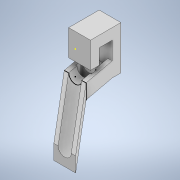
# Autodesk Inventor part: top_part
Saved by Autodesk Inventor 2021 (Build 250183000, 183)
## iProperties
Created: 2021-04-02
Part Number: top_part
Material: Generic
Document SubType Name: Modeling
Designer: Jawal
Density: 1 g/cm^3
Appearance: Default
Author: Jawal
Autodesk Inventor part; units mm, degrees
ref_plane "YZ Plane" through (0, 0, 0) normal (1, 0, 0) x (0, 1, 0)
ref_plane "XZ Plane" through (0, 0, 0) normal (0, 1, 0) x (-1, 0, 0)
ref_plane "XY Plane" through (0, 0, 0) normal (0, 0, 1) x (1, 0, 0)
sketch "Sketch1" plane through (0, 0, 0) normal (0, 0, 1) x (1, 0, 0)
  line L0 (-12.5, 12.5) -> (12.5, 12.5)
  line L1 (12.5, 12.5) -> (12.5, -37.5)
  line L2 (12.5, -37.5) -> (-12.5, -37.5)
  line L3 (-12.5, -37.5) -> (-12.5, 12.5)
  point P0 (0, 0)
  dimension "d0" = 25
  dimension "d1" = 50
  dimension "d2" = 12.5
  dimension "d3" = 12.5
  constraints: 8 end point, 2 parallel, 1 horizontal, 1 perpendicular
  measures "d0" distance of L0.start L0.end
  measures "d1" distance of L0.end L1.end
  measures "d2" distance from line of L1 point (0, 0)
  measures "d3" distance from line of point (0, 0) L0
extrude "Extrusion1" add sketch "Sketch1" along normal blind 10
sketch "Sketch2" plane through (0, 0, 0) normal (0, 0, -1) x (-1, 0, 0)
  circle A0 centre (0, -33) radius 1.5
  circle A1 centre (0, 0) radius 7.5
  dimension "d7" = 3
  dimension "d8" = 33
  dimension "d17" = 15
  constraints: 2 centre point, 1 coincident
  measures "d7" diameter of A0
  measures "d8" distance of A0.centre point (0, 0)
  measures "d17" diameter of A1
extrude "Extrusion2" add sketch "Sketch2" along normal blind 6 contours A0
sketch "Sketch3" plane through (0, 0, 10) normal (0, 0, 1) x (1, 0, 0)
  arc A0 (7.5, 0) -> (-7.5, 0) centre (0, 0) ccw
  line L0 (-7.5, 0) -> (-12.5, 0)
  line L1 (-12.5, 12.5) -> (-12.5, -37.5) projected
  line L2 (-12.5, 0) -> (-12.5, 12.5)
  line L3 (12.5, 12.5) -> (-12.5, 12.5) projected
  line L4 (12.5, 12.5) -> (12.5, 0)
  line L5 (12.5, -37.5) -> (12.5, 12.5) projected
  line L6 (7.5, 0) -> (12.5, 0)
  dimension "d11" = 15
  constraints: 8 end point, 2 point on circle, 2 point on line, 1 centre point, 1 coincident, 1 collinear, 1 horizontal, 1 perpendicular
  measures "d11" diameter of A0
extrude "Extrusion3" add sketch "Sketch3" along normal blind 15
sketch "Sketch4" plane through (0, 0, 25) normal (0, 0, 1) x (1, 0, 0)
  line L0 (-12.5, 12.5) -> (-12.5, 0) projected
  line L1 (-12.5, 12.5) -> (12.5, 12.5)
  line L2 (12.5, 12.5) -> (12.5, -17.5)
  line L3 (12.5, -17.5) -> (-12.5, -17.5)
  line L4 (-12.5, -17.5) -> (-12.5, 12.5)
  point P0 (0, 0)
  dimension "d14" = 25
  dimension "d21" = 30
  constraints: 8 end point, 2 parallel, 1 horizontal, 1 perpendicular
  measures "d14" distance of L2.end L3.end
  measures "d21" distance of L1.end L2.end
extrude "Extrusion4" add sketch "Sketch4" along normal blind 10
sketch "Sketch5" plane through (0, 0, 0) normal (0, 0, -1) x (-1, 0, 0)
  circle A0 centre (0, 0) radius 7.5
  dimension "d18" = 15
  constraints: 1 centre point, 1 coincident
  measures "d18" diameter of A0
extrude "Extrusion5" cut sketch "Sketch5" against normal blind 10
sketch "Sketch6" plane through (0, 0, 10) normal (0, 0, 1) x (1, 0, 0)
  line L0 (-12.5, -20.5) -> (-12.5, -37.5)
  line L1 (-12.5, -37.5) -> (12.5, -37.5) projected
  line L2 (-12.5, -37.5) -> (12.5, -37.5)
  line L3 (12.5, -37.5) -> (12.5, -20.5)
  line L4 (12.5, -37.5) -> (12.5, 0) projected
  arc A0 (-7.5, -20.5) -> (7.5, -20.5) centre (0, -20.5) ccw
  line L5 (-12.5, -20.5) -> (-7.5, -20.5)
  line L6 (7.5, -20.5) -> (12.5, -20.5)
  line L7 (-12.5, 0) -> (-12.5, -37.5) projected
  line L8 (-12.5, -29) -> (12.5, -29)
  point P0 (0, 0)
  dimension "d22" = 15
  dimension "d23" = 17
  dimension "d24" = 17
  constraints: 12 end point, 3 point on line, 2 horizontal, 2 point on circle, 1 centre point, 1 collinear, 1 perpendicular
  measures "d22" diameter of A0
  measures "d23" distance of L1.end L3.end
  measures "d24" distance of L0.start L0.end
ref_plane "Work Plane1" through (0, -37.5, 0) normal (-1, 0, 0) x (0, 0, 1)
sketch "Sketch8" plane through (0, -37.5, 0) normal (-1, 0, 0) x (0, 0, 1)
  line L0 (10, 0) -> (10, 37.5) projected
  line L1 (10, 8.5) -> (40, 1.574)
  line L2 (10, 8.5) -> (40.7891, 8.5) construction
  line L3 (0, 0) -> (10, 0) projected
  point P0 (0, 37.5)
  dimension "d26" = 13
  dimension "d27" = 8.5
  dimension "d32" = 30
  constraints: 4 end point, 1 equal length, 1 horizontal, 1 point on line
  measures "d26" angle of L1 L2
  measures "d27" distance between parallel lines of L3 L2
  measures "d32" distance from line of L1.end L0
sweep "Sweep1" add profiles "Sketch6" path "Sketch8" path curves L1
thread "Thread1"
sketch "Sketch9" plane through (-12.5, -44.426, 40) normal (0, 0, 1) x (1, 0, 0)
  point P0 (12.5, 44.426)
sketch "Sketch10" plane through (-12.5, -44.426, 40) normal (0, 0, 1) x (1, 0, 0)
  point P0 (12.5, 44.426)
ref_plane "Work Plane2" through (12.5, -44.426, 40) normal (0, -1, 0) x (1, 0, 0)
sketch "Sketch12" plane through (12.5, -44.426, 40) normal (0, -1, 0) x (1, 0, 0)
  line L0 (-3.5, -15.5) -> (-21.5, -15.5)
  line L1 (-21.5, -15.5) -> (-21.5, -9.5)
  line L2 (-21.5, -9.5) -> (-3.5, -9.5)
  line L3 (-3.5, -9.5) -> (-3.5, -15.5)
  line L4 (0, -30) -> (0, 0) projected
  point P0 (-12.5, -40)
  dimension "d33" = 18
  dimension "d34" = 6
  dimension "d35" = 3.5
  dimension "d36" = 14.5
  constraints: 8 end point, 1 horizontal, 1 parallel, 1 perpendicular
  measures "d33" distance of L1.end L2.end
  measures "d34" distance of L0.end L1.end
  measures "d35" distance between parallel lines of L4 L3
  measures "d36" distance from line of L4.start L0
extrude "Extrusion6" cut sketch "Sketch12" against normal blind 25
sketch "Sketch13" plane through (-12.5, -44.426, 40) normal (0, 0, 1) x (1, 0, 0)
  line L0 (5, 17) -> (0, 17) projected
  line L1 (5, 17) -> (0, 17)
  line L2 (0, 17) -> (0, 0) projected
  line L3 (0, 17) -> (0, 0)
  line L4 (0, 0) -> (25, 0) projected
  line L5 (0, 0) -> (25, 0)
  line L6 (25, 0) -> (25, 17) projected
  line L7 (25, 0) -> (25, 17)
  arc A0 (5, 17) -> (20, 17) centre (12.5, 17) ccw projected
  line L8 (25, 17) -> (20, 17)
  arc A1 (5, 17) -> (20, 17) centre (12.5, 17) ccw
  point P0 (12.5, 44.426)
  constraints: 10 end point, 2 collinear, 2 perpendicular, 2 point on circle, 1 centre point, 1 concentric, 1 horizontal
ref_plane "Work Plane3" through (-12.5, -44.426, 80) normal (0, 0, 1) x (1, 0, 0)
sketch "Sketch14" plane through (-12.5, -44.426, 80) normal (0, 0, 1) x (1, 0, 0)
  line L0 (28, -21.574) -> (28, -38.574)
  line L1 (28, -38.574) -> (53, -38.574)
  line L2 (53, -38.574) -> (53, -21.574)
  line L3 (53, -21.574) -> (48, -21.574)
  line L4 (28, -21.574) -> (33, -21.574)
  arc A0 (33, -21.574) -> (48, -21.574) centre (40.5, -21.574) ccw
  line L5 (5, 17) -> (0, 17) projected
  point P0 (12.5, 44.426)
  dimension "d40" = 17
  dimension "d41" = 25
  dimension "d42" = 5
  dimension "d43" = 5
  dimension "d45" = 15
  dimension "d46" = 38.574
  dimension "d47" = 28
  constraints: 10 end point, 3 perpendicular, 2 point on circle, 1 centre point, 1 horizontal, 1 vertical
  measures "d40" distance of L0.start L0.end
  measures "d41" distance of L0.end L1.end
  measures "d42" distance of L2.end L3.end
  measures "d43" distance of L0.start L4.end
  measures "d45" diameter of A0
  measures "d46" distance between parallel lines of L4 L5
  measures "d47" horizontal distance of L0.start L5.end
loft "Loft1" add profiles "Sketch14" section 1 edges at (-10, -27.426, 40) (-12.5, -35.926, 40) (0, -44.426, 40) (12.5, -35.926, 40) (10, -27.426, 40) (0, -34.926, 40)
equation "\"d2\" = 0.5 * d0"
equation "\"d24\" = d23"
body "Solid1"
